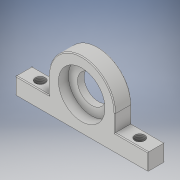
# Autodesk Inventor part: Chumacera (pieza extra)
Saved by Autodesk Inventor 2019.1 (Build 231200000, 200)
## iProperties
Created: 2024-03-28
Part Number: Chumacera (pieza extra)
Material: Generic
Document SubType Name: Modeling
Designer: clariheelen
Density: 1 g/cm^3
Appearance: Default
Author: clariheelen
Autodesk Inventor part; units mm, degrees
ref_plane "YZ Plane" through (0, 0, 0) normal (1, 0, 0) x (0, 1, 0)
ref_plane "XZ Plane" through (0, 0, 0) normal (0, 1, 0) x (-1, 0, 0)
ref_plane "XY Plane" through (0, 0, 0) normal (0, 0, 1) x (1, 0, 0)
sketch "Sketch6" plane through (0, 0, 0) normal (0, 0, 1) x (1, 0, 0)
  circle A0 centre (0, 0) radius 17.07
  circle A1 centre (0, 0) radius 28.07
  line L0 (-40, -40) -> (40, -40)
  line L1 (40, -40) -> (40, 0)
  line L2 (-40, 0) -> (-40, -40)
  circle A2 centre (0, 0) radius 40
  line L3 (-40, -40) -> (-80, -40)
  line L4 (-80, -40) -> (-80, -20)
  line L5 (-80, -20) -> (-40, -20)
  line L6 (-40, -20) -> (-40, -40)
  line L7 (40, -40) -> (80, -40)
  line L8 (80, -40) -> (80, -20)
  line L9 (80, -20) -> (40, -20)
  line L10 (40, -20) -> (40, -40)
  dimension "d29" = 34.14
  dimension "d30" = 56.14
  constraints: 22 end point, 5 parallel, 3 centre point, 3 coincident, 3 horizontal, 3 perpendicular, 2 point on circle
  measures "d29" diameter of A0
  measures "d30" diameter of A1
extrude "Extrusion5" add sketch "Sketch6" along normal blind 20 contours L2 A2 L0 | L3 L4 L5 L2 | A2 L1 L0 | A2 | L1 L9 L8 L7
sketch "Sketch7" plane through (0, 0, 0) normal (0, 0, -1) x (-1, 0, 0)
  circle A0 centre (0, 0) radius 17.07
  circle A1 centre (0, 0) radius 28.07
  dimension "d39" = 34.14
  dimension "d40" = 56.14
  constraints: 2 centre point, 2 coincident
  measures "d39" diameter of A0
  measures "d40" diameter of A1
extrude "Extrusion6" add sketch "Sketch7" against normal blind 8
sketch "Sketch8" plane through (-80, -20, 0) normal (0, 1, 0) x (1, 0, 0)
  line L0 (0, 0) -> (0, -20) projected
  line L1 (0, -20) -> (160, -20) projected
  line L2 (0, 0) -> (40, 0)
  line L3 (40, 0) -> (40, -20)
  line L4 (40, -20) -> (0, -20)
  line L5 (0, -20) -> (0, 0)
  circle A0 centre (20, -10) radius 6
  point P0 (80, 0)
  dimension "d44" = 12
  constraints: 8 end point, 2 parallel, 1 centre point, 1 horizontal, 1 perpendicular, 1 point on line
  measures "d44" diameter of A0
extrude "Extrusion7" cut sketch "Sketch8" against normal blind 20 contours A0
thread "Thread3" size "M12x1.75" class "6H" standard "ANSI Metric M Profile" full length
sketch "Sketch9" plane through (40, -20, 0) normal (0, 1, 0) x (1, 0, 0)
  line L0 (0, 0) -> (0, -20) projected
  line L1 (40, 0) -> (40, -20) projected
  line L2 (0, 0) -> (40, 0)
  line L3 (40, 0) -> (40, -20)
  line L4 (40, -20) -> (0, -20)
  line L5 (0, -20) -> (0, 0)
  circle A0 centre (20, -10) radius 6
  point P0 (-40, 0)
  dimension "d49" = 12
  constraints: 8 end point, 2 parallel, 1 centre point, 1 horizontal, 1 perpendicular
  measures "d49" diameter of A0
extrude "Extrusion8" cut sketch "Sketch9" against normal blind 20 contours A0
thread "Thread4" size "M12x1.75" class "6H" standard "ANSI Metric M Profile" full length
fillet "Fillet3" radius 1 15 edges at (-60, -20, 20) (-60, -20, 0) (-80, -20, 10) (-80, -30, 0) (-80, -30, 20) (60, -20, 20) (60, -20, 0) (80, -30, 20) (80, -30, 0) (0, 40, 20) (-40, -10, 20) (40, -10, 20) (0, 40, 0) (-40, -10, 0) (40, -10, 0)
body "Solid2"
